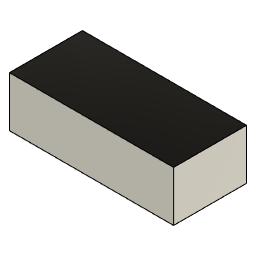
psu_board_step (Autodesk Fusion 360 archive; units mm, degrees)
design "電圧計"
Autodesk Fusion 360 part; units mm, degrees
sketch "スケッチ1" plane through (0, 0, 0) normal (0, 0, 1) x (1, 0, 0)
  line L0 (0, 0) -> (22.86, 0)
  line L1 (22.86, 0) -> (22.86, 10.16)
  line L2 (22.86, 10.16) -> (0, 10.16)
  line L3 (0, 10.16) -> (0, 0)
  dimension "d1" = 22.86
  dimension "d2" = 10.16
  constraint horizontal L0
  constraint vertical L1
  constraint horizontal L2
  constraint vertical L3
  constraint coincident L0.start L3.end
  measures "d1" distance of L0.start L0.end
  measures "d2" distance of L0.start L2.end
extrude "押し出し1" add sketch "スケッチ1" along normal blind 7

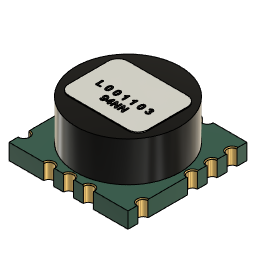
design "ムラタ　デコデコ"
Autodesk Fusion 360 part; units mm, degrees
sketch "スケッチ1" plane through (0, 0, 0) normal (0, 0, 1) x (1, 0, 0)
  line L0 (0, 0) -> (12, 0)
  line L1 (12, 0) -> (12, 12)
  line L2 (12, 12) -> (0, 12)
  line L3 (0, 12) -> (0, 0)
  dimension "d1" = 12
  dimension "d2" = 12
  constraint horizontal L0
  constraint vertical L1
  constraint horizontal L2
  constraint vertical L3
  constraint coincident L0.start L3.end
  measures "d1" distance of L0.start L0.end
  measures "d2" distance of L0.start L2.end
extrude "押し出し1" add sketch "スケッチ1" along normal blind 1.6
sketch "スケッチ2" plane through (0, 0, 1.6) normal (0, 0, 1) x (-1, 0, 0)
  line L0 (0, -12) -> (0, 0)
  line L1 (0, 0) -> (-12, 0)
  line L2 (-12, 0) -> (-12, -12)
  line L3 (-12, -12) -> (0, -12)
  circle A0 centre (-6, -6) radius 5.25
  dimension "d5" = 10.5
  measures "d5" diameter of A0
extrude "押し出し2" add sketch "スケッチ2" along normal blind 4 contours A0
sketch "スケッチ3" plane through (0, 0, 1.6) normal (0, 0, 1) x (-1, 0, 0)
  circle A0 centre (-6, -6) radius 5.25
  line L0 (0, -12) -> (0, 0)
  line L1 (0, 0) -> (-12, 0)
  line L2 (-12, 0) -> (-12, -12)
  line L3 (-12, -12) -> (0, -12)
  line L4 (-6, -12) -> (-8, -12)
  line L5 (-6, -12) -> (-4, -12)
  circle A1 centre (-8, -12) radius 0.5
  circle A2 centre (-4, -12) radius 0.5
  circle A3 centre (-6, -12) radius 0.5
  line L6 (-6, 0) -> (-8, 0)
  line L7 (-6, 0) -> (-4, 0)
  circle A4 centre (-8, 0) radius 0.5
  circle A5 centre (-6, 0) radius 0.5
  circle A6 centre (-4, 0) radius 0.5
  line L8 (-12, 0) -> (-12, -1.5)
  line L9 (0, 0) -> (0, -1.5)
  line L10 (0, -12) -> (0, -10.5)
  line L11 (0, -10.5) -> (0, -8.5)
  line L12 (0, -8.5) -> (0, -6.5)
  line L13 (0, -6.5) -> (0, -4.5)
  line L14 (-12, -12) -> (-12, -10.5)
  line L15 (-12, -10.5) -> (-12, -8.5)
  line L16 (-12, -8.5) -> (-12, -6.5)
  line L17 (-12, -6.5) -> (-12, -4.5)
  circle A7 centre (-12, -4.5) radius 0.5
  circle A8 centre (-12, -6.5) radius 0.5
  circle A9 centre (-12, -8.5) radius 0.5
  circle A10 centre (-12, -10.5) radius 0.5
  circle A11 centre (0, -10.5) radius 0.5
  circle A12 centre (0, -8.5) radius 0.5
  circle A13 centre (0, -6.5) radius 0.5
  circle A14 centre (0, -1.5) radius 0.5
  circle A15 centre (-12, -1.5) radius 0.5
  dimension "d8" = 2
  dimension "d9" = 2
  dimension "d10" = 1
  dimension "d11" = 1
  dimension "d12" = 1
  dimension "d13" = 2
  dimension "d14" = 2
  dimension "d15" = 1
  dimension "d16" = 1
  dimension "d17" = 1
  dimension "d18" = 1.5
  dimension "d19" = 1.5
  dimension "d20" = 1.5
  dimension "d21" = 2
  dimension "d22" = 2
  dimension "d23" = 2
  dimension "d24" = 1.5
  dimension "d25" = 2
  dimension "d26" = 2
  dimension "d27" = 2
  dimension "d28" = 1
  dimension "d29" = 1
  dimension "d30" = 1
  dimension "d31" = 1
  dimension "d32" = 1
  dimension "d33" = 1
  dimension "d34" = 1
  dimension "d35" = 1
  dimension "d36" = 1
  constraint midpoint L3 L4.start
  constraint parallel L3 L4
  constraint parallel L3 L5
  constraint coincident L4.end A1.centre
  constraint coincident L5.end A2.centre
  constraint coincident L4.start L5.start
  constraint midpoint L1 L6.start
  constraint perpendicular L0 L6
  constraint perpendicular L0 L7
  constraint coincident L6.end A4.centre
  constraint coincident L6.start L7.start
  constraint coincident L7.end A6.centre
  constraint coincident L1.end L2.start
  constraint perpendicular L1 L8
  constraint coincident L0.end L1.start
  constraint perpendicular L1 L9
  constraint coincident L0.start L3.end
  constraint perpendicular L3 L10
  constraint parallel L0 L11
  constraint parallel L0 L12
  constraint parallel L0 L13
  constraint coincident L2.end L3.start
  constraint perpendicular L3 L14
  constraint perpendicular L3 L15
  constraint parallel L2 L16
  constraint parallel L2 L17
  constraint coincident L17.end A7.centre
  constraint coincident L16.end L17.start
  constraint coincident L15.end L16.start
  constraint coincident L14.end L15.start
  constraint coincident L10.end L11.start
  constraint coincident L11.end L12.start
  constraint coincident L12.end L13.start
  constraint coincident L9.end A14.centre
  constraint coincident L8.end A15.centre
  measures "d8" distance of L4.start L4.end
  measures "d9" distance of L4.start L5.end
  measures "d10" diameter of A1
  measures "d11" diameter of A2
  measures "d12" diameter of A3
  measures "d13" distance of L6.start L6.end
  measures "d14" distance of L6.start L7.end
  measures "d15" diameter of A4
  measures "d16" diameter of A5
  measures "d17" diameter of A6
  measures "d18" distance of L1.end L8.end
  measures "d19" distance of L0.end L9.end
  measures "d20" distance of L0.start L10.end
  measures "d21" distance of L10.end L11.end
  measures "d22" distance of L11.end L12.end
  measures "d23" distance of L12.end L13.end
  measures "d24" distance of L2.end L14.end
  measures "d25" distance of L14.end L15.end
  measures "d26" distance of L15.end L16.end
  measures "d27" distance of L16.end L17.end
  measures "d28" diameter of A7
  measures "d29" diameter of A8
  measures "d30" diameter of A9
  measures "d31" diameter of A10
  measures "d32" diameter of A11
  measures "d33" diameter of A12
  measures "d34" diameter of A13
  measures "d35" diameter of A14
  measures "d36" diameter of A15
extrude "押し出し3" cut sketch "スケッチ3" against normal blind 2.5 contours L0 L10 L11 A11 | L3 L5 A2 | L0 L11 L12 A12 | L3 L4 L5 A3 | L0 L12 L13 A13 | L3 L4 A1 | L0 L9 A14 | L2 L14 L15 A10 | L2 L15 L16 A9 | L1 L7 A6 | L2 L16 L17 A8 | L1 L6 L7 A5 | L1 L6 A4 | L2 L8 A15 picked at (-0.2072, -10.7599) picked at (-3.7401, -11.7928) picked at (-0.2072, -8.7599) picked at (-6.2599, -11.7928) picked at (-0.3324, -6.5) picked at (-8.2599, -11.7928) picked at (-0.2072, -1.7599) picked at (-11.7082, -10.6593) picked at (-11.7082, -8.6593) picked at (-4.3315, -0.0248) picked at (-11.6885, -6.6162) picked at (-6.3315, -0.0248) picked at (-8.3315, -0.0248) picked at (-11.6885, -1.6162)
sketch "スケッチ4" plane through (0, 0, 5.6) normal (0, 0, 1) x (-1, 0, 0)
  circle A0 centre (-6, -6) radius 5.25
  line L0 (-6, -6) -> (-9, -6)
  line L1 (-9, -6) -> (-9, -8)
  line L2 (-9, -8) -> (-6, -8)
  line L3 (-6, -8) -> (-6, -6)
  line L4 (-6, -6) -> (-9, -6)
  line L5 (-9, -6) -> (-9, -4)
  line L6 (-9, -4) -> (-6, -4)
  line L7 (-6, -4) -> (-6, -6)
  line L8 (-6, -6) -> (-3, -6)
  line L9 (-3, -6) -> (-3, -4)
  line L10 (-3, -4) -> (-6, -4)
  line L11 (-6, -4) -> (-6, -6)
  line L12 (-3, -6) -> (-6, -6)
  line L13 (-6, -6) -> (-6, -8)
  line L14 (-6, -8) -> (-3, -8)
  line L15 (-3, -8) -> (-3, -6)
  line L16 (-2.5, -8.5) -> (-9.5, -8.5)
  line L17 (-9.5, -8.5) -> (-9.5, -3.5)
  line L18 (-9.5, -3.5) -> (-2.5, -3.5)
  line L19 (-2.5, -3.5) -> (-2.5, -8.5)
  line L20 (-2, -9) -> (-10, -9)
  line L21 (-10, -9) -> (-10, -3)
  line L22 (-10, -3) -> (-2, -3)
  line L23 (-2, -3) -> (-2, -9)
  constraint horizontal L0
  constraint vertical L1
  constraint horizontal L2
  constraint vertical L3
  constraint coincident A0.centre L0.start
  constraint horizontal L4
  constraint vertical L5
  constraint horizontal L6
  constraint vertical L7
  constraint horizontal L8
  constraint vertical L9
  constraint horizontal L10
  constraint vertical L11
  constraint horizontal L12
  constraint vertical L13
  constraint horizontal L14
  constraint vertical L15
  constraint horizontal L16
  constraint vertical L17
  constraint horizontal L18
  constraint vertical L19
  constraint horizontal L20
  constraint vertical L21
  constraint horizontal L22
  constraint vertical L23
extrude "押し出し4" add sketch "スケッチ4" along normal blind 0.1 contours L0 L1 L2 L3 L4 L13 | L3 L8 L12 L13 L14 L15 | L0 L4 L5 L6 L7 L11 | L7 L8 L9 L10 L11 L12 | L16 L17 L18 L19 | L20 L21 L22 L23
fillet "フィレット1" radius 1 4 edges at (10, 3, 5.65) (10, 9, 5.65) (2, 3, 5.65) (2, 9, 5.65)
sketch "スケッチ5" plane through (0, 0, 5.7) normal (0, 0, 1) x (-1, 0, 0)
  arc A0 (-3, -9) -> (-2, -8) centre (-3, -8) ccw
  line L0 (-2, -8) -> (-2, -4)
  arc A1 (-2, -4) -> (-3, -3) centre (-3, -4) ccw
  line L1 (-3, -3) -> (-9, -3)
  arc A2 (-9, -3) -> (-10, -4) centre (-9, -4) ccw
  line L2 (-10, -4) -> (-10, -8)
  arc A3 (-10, -8) -> (-9, -9) centre (-9, -8) ccw
  line L3 (-9, -9) -> (-3, -9)
  line L4 (-2.7649, -3.5228) -> (-9.3213, -3.5088) construction
  line L5 (-9.3213, -3.5088) -> (-9.3267, -6.028) construction
  line L6 (-9.3267, -6.028) -> (-2.7703, -6.042) construction
  line L7 (-2.7703, -6.042) -> (-2.7649, -3.5228) construction
  dimension "d43" = 0.7
  text T0 "L 0 0 1 1 0 3\n94NN" font "Arial" height 0.7 bold align centre top in box 6.5564 x 2.5192 at (-2.7649, -3.5228) x (-0.999998, 0.002128) y (-0.002128, -0.999998) spacing 1 kerned
extrude "押し出し5" cut sketch "スケッチ5" against normal blind 0.01 text T0
fillet "フィレット2" radius 0.1 14 edges at (4, 0.5, 1.6) (6, 0.5, 1.6) (8, 0.5, 1.6) (0.5, 1.5, 1.6) (0.5, 6.5, 1.6) (0.5, 8.5, 1.6) (0.5, 10.5, 1.6) (4, 11.5, 1.6) (6, 11.5, 1.6) (8, 11.5, 1.6) (11.5, 10.5, 1.6) (11.5, 8.5, 1.6) (11.5, 6.5, 1.6) (11.5, 1.5, 1.6)
